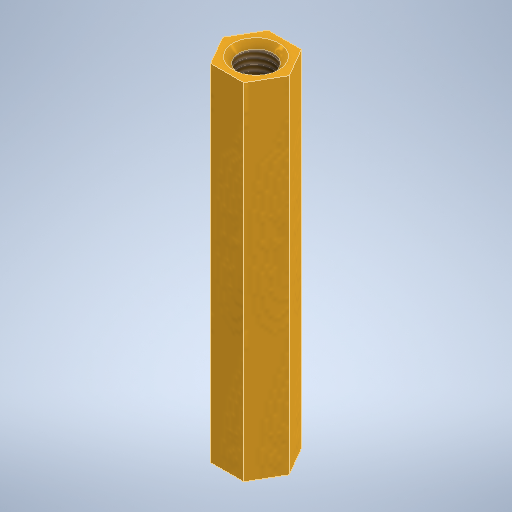
# Autodesk Inventor part: suporte
Saved by Autodesk Inventor 2025.1 (Build 291241000, 241)
## iProperties
Created: 2024-09-05
Part Number: suporte
Material: Latão, amarelo macio, soldado
Document SubType Name: Modeling
Designer: Célio
Density: 8.5 g/cm^3
Appearance: Latão - Soldado
Author: Célio
Autodesk Inventor part; units mm, degrees
ref_plane "YZ Plane" through (0, 0, 0) normal (1, 0, 0) x (0, 1, 0)
ref_plane "XZ Plane" through (0, 0, 0) normal (0, 1, 0) x (-1, 0, 0)
ref_plane "XY Plane" through (0, 0, 0) normal (0, 0, 1) x (1, 0, 0)
sketch "Esboço1" plane through (0, 0, 0) normal (0, 1, 0) x (-1, 0, 0)
  line L0 (-1.4434, -2.5) -> (-2.8868, 0)
  line L1 (-2.8868, 0) -> (-1.4434, 2.5)
  line L2 (-1.4434, 2.5) -> (1.4434, 2.5)
  line L3 (1.4434, 2.5) -> (2.8868, 0)
  line L4 (2.8868, 0) -> (1.4434, -2.5)
  line L5 (1.4434, -2.5) -> (-1.4434, -2.5)
  circle A0 centre (0, 0) radius 1.5
  point P0 (0, -2.5)
  constraints: 12 end point, 1 centre point, 1 coincident, 1 midpoint, 13 other
extrude "Extrusão1" add sketch "Esboço1" along normal blind 30
chamfer "Chanfro1" distance 0.5 angle 45 2 edges at (1.5, 30, 0) (1.5, 0, 0)
thread "Rosca1" size "M3x0.5" class "6H" standard "ANSI Metric M Profile" full length
